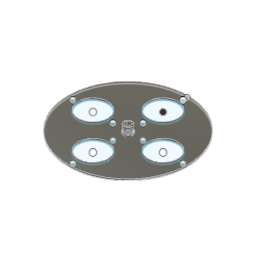
filterwheel v7 (Autodesk Fusion 360 design; units mm, degrees)
Autodesk Fusion 360 part; units mm, degrees
note: some values were not read from the file. Set by a fixed rule: which sketch regions a step uses.
sketch "Sketch1" plane through (0, 0, 0) normal (0, 0, 1) x (1, 0, 0)
  circle A0 centre (0, 0) radius 2.5
  circle A1 centre (0, 0) radius 1.775
  circle A2 centre (0, 0) radius 3.5
  line L0 (1.775, 0) -> (1.775, 3.0165)
  line L1 (1.775, 0) -> (1.775, -3.0165)
  circle A3 centre (0, 0) radius 48.5
  circle A4 centre (0, 44.6993) radius 1.45
  circle A5 centre (0, 44.6993) radius 1.45
  circle A6 centre (0, 12.1993) radius 1.45
  circle A7 centre (0, 28.4493) radius 12
  circle A8 centre (-44.6993, 0) radius 1.45
  circle A9 centre (-28.4493, 0) radius 12
  circle A10 centre (-12.1993, 0) radius 1.45
  circle A11 centre (0, -44.6993) radius 1.45
  circle A12 centre (0, -28.4493) radius 12
  circle A13 centre (0, -12.1993) radius 1.45
  circle A14 centre (44.6993, 0) radius 1.45
  circle A15 centre (28.4493, 0) radius 12
  circle A16 centre (12.1993, 0) radius 1.45
  point P0 (0, 47.6993)
  point P1 (0, 28.4493)
  dimension "d1" = 5
  dimension "d3" = 3.55
  dimension "d4" = 7
  dimension "d5" = 97
  dimension "d7" = 2.9
  dimension "d8" = 32.5
  dimension "d9" = 2.9
  dimension "d10" = 2.9
  dimension "d11" = 24
  dimension "d13" = 360
  constraint coincident A0.centre A1.centre
  constraint concentric A0 A1
  constraint concentric A0 A2
  constraint coincident A1 L0.start
  constraint coincident A2 L0.end
  constraint tangent A1 L0
  constraint vertical L0
  constraint coincident A2 L1.end
  constraint tangent A1 L1
  constraint concentric A1 A3
  constraint coincident P1 A7.centre
  measures "d1" diameter of A0
  measures "d3" diameter of A1
  measures "d4" diameter of A2
  measures "d5" diameter of A3
  measures "d7" diameter of A4
  measures "d8" distance of A4.centre A6.centre
  measures "d9" diameter of A5
  measures "d10" diameter of A6
  measures "d11" diameter of A7
extrude "Extrude4" add sketch "Sketch1" along normal blind 6 contours A0 L0 L1 | A0 A2 L0 L1 | A0 A2 L0 L1 picked at (2.2513, 0.1082) makes body 1
extrude "Extrude3" add sketch "Sketch1" along normal blind 2 separate body contours A0 L0 L1 | A0 A2 L0 L1 | A0 A2 L0 L1 picked at (2.2513, 0.1082) makes body 2
extrude "Extrude5" add sketch "Sketch1" along normal blind 1.5 contours A3 bodies 1 2
